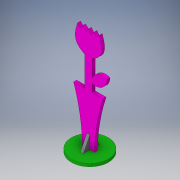
# Autodesk Inventor part: present_8_march
Saved by Autodesk Inventor 2019 (Build 230136000, 136)
## iProperties
Created: 2020-02-28
Part Number: present_8_march
Material: Типовые
Document SubType Name: Modeling
Designer: Alexander
Density: 1 g/cm^3
Appearance: По умолчанию
Author: Alexander
Autodesk Inventor part; units mm, degrees
ref_plane "YZ Plane" through (0, 0, 0) normal (1, 0, 0) x (0, 1, 0)
ref_plane "XZ Plane" through (0, 0, 0) normal (0, 1, 0) x (-1, 0, 0)
ref_plane "XY Plane" through (0, 0, 0) normal (0, 0, 1) x (1, 0, 0)
sketch "Эскиз2" plane through (0, 0, 0) normal (0, 1, 0) x (-1, 0, 0)
  circle A0 centre (0, 0) radius 25
  dimension "d13" = 50
  constraints: 1 centre point, 1 coincident
  measures "d13" diameter of A0
extrude "Выдавливание2" add sketch "Эскиз2" along normal blind 4
sketch "Эскиз3" plane through (0, 0, 0) normal (0, 0, 1) x (1, 0, 0)
  line L0 (-5, 73) -> (-20, 73)
  line L1 (5, 73) -> (20, 73)
  arc A0 (-8, 3) -> (-20, 73) centre (-241.9644, -1.0796) ccw
  arc A1 (20, 73) -> (8, 3) centre (241.9644, -1.0796) ccw
  line L2 (20, 73) -> (20, 113) construction
  line L3 (20, 113) -> (-20, 113) construction
  line L4 (0, 73) -> (5, 73) construction
  line L5 (-5, 73) -> (-5, 113)
  line L6 (0, 145) -> (-19, 145) construction
  line L7 (0, 145) -> (19, 145) construction
  line L8 (-19, 145) -> (-19, 113) construction
  line L9 (19, 145) -> (19, 113) construction
  spline S0 degree 4 poles (-5, 113) (-14.4011, 117.5623) (-19, 126.1751) (-18.0742, 132.6347) (-17.0609, 137.5744) (-14.6544, 145) knots 1 1 1 1 1 2 3 3 3 3 3
  spline S1 degree 4 poles (5, 113) (14.4011, 117.5623) (19, 126.1751) (18.0742, 132.6347) (17.0609, 137.5744) (14.6544, 145) knots 1 1 1 1 1 2 3 3 3 3 3
  line L10 (0, 145) -> (-3.1568, 140.6381)
  line L11 (-3.1568, 140.6381) -> (-8, 145)
  line L12 (-8, 145) -> (-11.012, 140.2331)
  line L13 (-11.012, 140.2331) -> (-14.6544, 145)
  line L14 (0, 145) -> (3.8002, 140.0266)
  line L15 (3.8002, 140.0266) -> (7.3995, 145)
  line L16 (7.3995, 145) -> (10.7295, 140.642)
  line L17 (10.7295, 140.642) -> (14.6544, 145)
  line L18 (-8, 3) -> (-6, 3)
  line L19 (8, 3) -> (6, 3)
  arc A2 (5, 83.5644) -> (25.2233, 98.6424) centre (9.5, 98.63) ccw
  arc A3 (25.2233, 98.6424) -> (5, 90.0664) centre (19.4936, 84.0211) ccw
  line L20 (5, 73) -> (5, 83.5644)
  line L21 (5, 90.0664) -> (5, 113)
  line L22 (-6, 3) -> (-6, 0)
  line L23 (-6, 0) -> (-2, 0)
  line L24 (-2, 0) -> (-2, 3)
  line L25 (6, 3) -> (6, 0)
  line L26 (6, 0) -> (2, 0)
  line L27 (2, 0) -> (2, 3)
  line L28 (-2, 3) -> (2, 3)
  point P0 (0, 0)
  point P1 (-9.2058, 115.3367)
  point P2 (-12.1464, 117.5105)
  point P3 (-15.5923, 121.4538)
  point P4 (-17.176, 125.0324)
  point P5 (-17.792, 128.3904)
  point P6 (-17.5188, 134.5733)
  point P7 (9.2058, 115.3367)
  point P8 (12.1464, 117.5105)
  point P9 (15.5923, 121.4538)
  point P10 (17.176, 125.0324)
  point P11 (17.792, 128.3904)
  point P12 (17.5188, 134.5733)
  dimension "d18" = 145
  dimension "d20" = 20
  dimension "d21" = 20
  dimension "d23" = 234
  dimension "d24" = 234
  dimension "d25" = 40
  dimension "d26" = 5
  dimension "d27" = 19
  dimension "d28" = 19
  dimension "d31" = 2
  dimension "d42" = 2
  dimension "d43" = 4
  dimension "d44" = 4
  constraints: 58 end point, 8 point on circle, 6 perpendicular, 6 point on line, 4 centre point, 4 horizontal, 3 parallel, 2 vertical, 16 other
  measures "d18" distance of point (0, 0) L6.start
  measures "d20" distance of L4.start L0.end
  measures "d21" distance of L4.start L1.end
  measures "d23" radius of A0
  measures "d24" radius of A1
  measures "d25" distance of L1.end L2.end
  measures "d26" distance of L4.start L1.start
  measures "d27" distance of L6.start L6.end
  measures "d28" distance of L6.start L7.end
  measures "d31" distance of L18.start L18.end
  measures "d42" distance of L19.start L19.end
  measures "d43" distance of L22.end L23.end
  measures "d44" distance of L25.end L26.end
extrude "Выдавливание4" add sketch "Эскиз3" along normal mid plane 4 separate body
sketch "Эскиз4" plane through (0, 0, 0) normal (1, 0, 0) x (0, 1, 0)
  line L0 (145, -2) -> (3, -2) construction
  line L1 (3, -25) -> (0, -25) construction
  line L2 (3, 2) -> (145, 2) construction
  line L3 (145, 2) -> (145, -2) construction
  line L4 (23, -1.5) -> (23, 1.5)
  line L5 (3, 2) -> (73, 2) projected
  line L6 (3, 11.5) -> (23, 1.5)
  line L7 (3, -11.5) -> (23, -1.5)
  line L8 (3, -2) -> (3, 2)
  line L9 (3, -11.5) -> (3, -7.5)
  line L10 (3, -7.5) -> (0, -7.5)
  line L11 (0, -7.5) -> (0, -3.5)
  line L12 (0, -3.5) -> (3, -3.5)
  line L13 (3, 11.5) -> (3, 7.5)
  line L14 (3, 7.5) -> (0, 7.5)
  line L15 (0, 7.5) -> (0, 3.5)
  line L16 (0, 3.5) -> (3, 3.5)
  line L17 (3, 3.5) -> (3, -3.5)
  point P0 (0, 0)
  dimension "d46" = 4
  dimension "d47" = 4
  dimension "d48" = 4
  dimension "d49" = 4
  constraints: 34 end point, 2 perpendicular, 1 other
  measures "d46" distance of L7.start L9.end
  measures "d47" distance of L10.end L11.end
  measures "d48" distance of L6.start L13.end
  measures "d49" distance of L14.end L15.end
extrude "Выдавливание5" add sketch "Эскиз4" along normal mid plane 4 separate body
combine bodies "Комбинировать4" operation type subtract main body 2 bodies to subtract 3 keep tools yes
combine bodies "Комбинировать5" operation type subtract main body 1 bodies to subtract 3 keep tools yes
combine bodies "Комбинировать6" operation type subtract main body 1 bodies to subtract 2 keep tools yes
equation "\"d14\" = толщина"
equation "\"d43\" = толщина"
equation "\"d44\" = толщина"
equation "\"d33\" = толщина"
equation "\"d47\" = толщина"
equation "\"d49\" = толщина"
equation "\"d40\" = толщина"
equation "\"толщина\" = 4"
